Autodesk Inventor part; units mm, degrees
(part 2 of 4)
  spline S285 degree 3 poles (-158.7452, 2.7796) (-159.3519, 3.3863) (-159.5334, 4.2987) (-159.205, 5.0914) knots 0 0 0 0 1 1 1 1 construction
  spline S286 degree 3 poles (-159.205, 5.0914) (-158.8767, 5.8841) (-158.1032, 6.4009) (-157.2452, 6.4009) knots 0 0 0 0 1 1 1 1 construction
  arc A68 (-155.1239, 4.2796) -> (-157.2452, 6.4009) centre (-157.2452, 4.2796) ccw construction
  spline S287 degree 3 poles (-145.4719, 23.3296) (-145.4719, 22.4716) (-145.9887, 21.6981) (-146.7814, 21.3698) knots 0 0 0 0 1 1 1 1 construction
  spline S288 degree 3 poles (-146.7814, 21.3698) (-147.5741, 21.0414) (-148.4865, 21.2229) (-149.0932, 21.8296) knots 0 0 0 0 1 1 1 1 construction
  spline S289 degree 3 poles (-149.0932, 21.8296) (-149.6999, 22.4363) (-149.8814, 23.3487) (-149.553, 24.1414) knots 0 0 0 0 1 1 1 1 construction
  spline S290 degree 3 poles (-149.553, 24.1414) (-149.2247, 24.9341) (-148.4512, 25.4509) (-147.5932, 25.4509) knots 0 0 0 0 1 1 1 1 construction
  arc A69 (-145.4719, 23.3296) -> (-147.5932, 25.4509) centre (-147.5932, 23.3296) ccw construction
  spline S291 degree 3 poles (-136.0739, 4.2796) (-136.0739, 3.4216) (-136.5907, 2.6481) (-137.3834, 2.3198) knots 0 0 0 0 1 1 1 1 construction
  spline S292 degree 3 poles (-137.3834, 2.3198) (-138.1761, 1.9914) (-139.0885, 2.1729) (-139.6952, 2.7796) knots 0 0 0 0 1 1 1 1 construction
  spline S293 degree 3 poles (-139.6952, 2.7796) (-140.3019, 3.3863) (-140.4834, 4.2987) (-140.155, 5.0914) knots 0 0 0 0 1 1 1 1 construction
  spline S294 degree 3 poles (-140.155, 5.0914) (-139.8267, 5.8841) (-139.0532, 6.4009) (-138.1952, 6.4009) knots 0 0 0 0 1 1 1 1 construction
  arc A70 (-136.0739, 4.2796) -> (-138.1952, 6.4009) centre (-138.1952, 4.2796) ccw construction
  spline S295 degree 3 poles (-140.6459, -33.8204) (-140.6459, -34.6784) (-141.1627, -35.4519) (-141.9554, -35.7802) knots 0 0 0 0 1 1 1 1 construction
  spline S296 degree 3 poles (-141.9554, -35.7802) (-142.7481, -36.1086) (-143.6605, -35.9271) (-144.2672, -35.3204) knots 0 0 0 0 1 1 1 1 construction
  spline S297 degree 3 poles (-144.2672, -35.3204) (-144.8739, -34.7137) (-145.0554, -33.8013) (-144.727, -33.0086) knots 0 0 0 0 1 1 1 1 construction
  spline S298 degree 3 poles (-144.727, -33.0086) (-144.3987, -32.2159) (-143.6252, -31.6991) (-142.7672, -31.6991) knots 0 0 0 0 1 1 1 1 construction
  arc A71 (-140.6459, -33.8204) -> (-142.7672, -31.6991) centre (-142.7672, -33.8204) ccw construction
  spline S299 degree 3 poles (-131.2479, -14.7704) (-131.2479, -15.6284) (-131.7647, -16.4019) (-132.5574, -16.7302) knots 0 0 0 0 1 1 1 1 construction
  spline S300 degree 3 poles (-132.5574, -16.7302) (-133.3501, -17.0586) (-134.2625, -16.8771) (-134.8692, -16.2704) knots 0 0 0 0 1 1 1 1 construction
  spline S301 degree 3 poles (-134.8692, -16.2704) (-135.4759, -15.6637) (-135.6574, -14.7513) (-135.329, -13.9586) knots 0 0 0 0 1 1 1 1 construction
  spline S302 degree 3 poles (-135.329, -13.9586) (-135.0007, -13.1659) (-134.2272, -12.6491) (-133.3692, -12.6491) knots 0 0 0 0 1 1 1 1 construction
  arc A72 (-131.2479, -14.7704) -> (-133.3692, -12.6491) centre (-133.3692, -14.7704) ccw construction
  spline S303 degree 3 poles (-121.5959, -33.8204) (-121.5959, -34.6784) (-122.1127, -35.4519) (-122.9054, -35.7802) knots 0 0 0 0 1 1 1 1 construction
  spline S304 degree 3 poles (-122.9054, -35.7802) (-123.6981, -36.1086) (-124.6105, -35.9271) (-125.2172, -35.3204) knots 0 0 0 0 1 1 1 1 construction
  spline S305 degree 3 poles (-125.2172, -35.3204) (-125.8239, -34.7137) (-126.0054, -33.8013) (-125.677, -33.0086) knots 0 0 0 0 1 1 1 1 construction
  spline S306 degree 3 poles (-125.677, -33.0086) (-125.3487, -32.2159) (-124.5752, -31.6991) (-123.7172, -31.6991) knots 0 0 0 0 1 1 1 1 construction
  arc A73 (-121.5959, -33.8204) -> (-123.7172, -31.6991) centre (-123.7172, -33.8204) ccw construction
  arc A74 (-102.5459, -33.8204) -> (-104.6672, -31.6991) centre (-104.6672, -33.8204) ccw construction
  spline S307 degree 3 poles (-102.5459, -33.8204) (-102.5459, -34.6784) (-103.0627, -35.4519) (-103.8554, -35.7802) knots 0 0 0 0 1 1 1 1 construction
  spline S308 degree 3 poles (-103.8554, -35.7802) (-104.6481, -36.1086) (-105.5605, -35.9271) (-106.1672, -35.3204) knots 0 0 0 0 1 1 1 1 construction
  spline S309 degree 3 poles (-106.1672, -35.3204) (-106.7739, -34.7137) (-106.9554, -33.8013) (-106.627, -33.0086) knots 0 0 0 0 1 1 1 1 construction
  spline S310 degree 3 poles (-106.627, -33.0086) (-106.2987, -32.2159) (-105.5252, -31.6991) (-104.6672, -31.6991) knots 0 0 0 0 1 1 1 1 construction
  spline S311 degree 3 poles (-112.1979, -14.7704) (-112.1979, -15.6284) (-112.7147, -16.4019) (-113.5074, -16.7302) knots 0 0 0 0 1 1 1 1 construction
  spline S312 degree 3 poles (-113.5074, -16.7302) (-114.3001, -17.0586) (-115.2125, -16.8771) (-115.8192, -16.2704) knots 0 0 0 0 1 1 1 1 construction
  spline S313 degree 3 poles (-115.8192, -16.2704) (-116.4259, -15.6637) (-116.6074, -14.7513) (-116.279, -13.9586) knots 0 0 0 0 1 1 1 1 construction
  spline S314 degree 3 poles (-116.279, -13.9586) (-115.9507, -13.1659) (-115.1772, -12.6491) (-114.3192, -12.6491) knots 0 0 0 0 1 1 1 1 construction
  arc A75 (-112.1979, -14.7704) -> (-114.3192, -12.6491) centre (-114.3192, -14.7704) ccw construction
  line L28 (-145.8754, -43.9454) -> (-139.8754, -43.9454) construction
  line L29 (-139.8754, -43.9454) -> (-139.8754, -58.9454) construction
  line L30 (-139.8754, -58.9454) -> (-145.8754, -58.9454) construction
  line L31 (-145.8754, -58.9454) -> (-145.8754, -43.9454) construction
  spline S315 degree 3 poles (-134.5894, 49.9986) (-135.3821, 49.6702) (-136.2945, 49.8517) (-136.9012, 50.4584) knots 0 0 0 0 1 1 1 1 construction
  spline S316 degree 3 poles (-136.9012, 50.4584) (-137.5079, 51.0651) (-137.6894, 51.9775) (-137.361, 52.7702) knots 0 0 0 0 1 1 1 1 construction
  spline S317 degree 3 poles (-137.361, 52.7702) (-137.0327, 53.5629) (-136.2592, 54.0797) (-135.4012, 54.0797) knots 0 0 0 0 1 1 1 1 construction
  arc A76 (-133.2799, 51.9584) -> (-135.4012, 54.0797) centre (-135.4012, 51.9584) ccw construction
  spline S318 degree 3 poles (-133.2799, 51.9584) (-133.2799, 51.1004) (-133.7967, 50.3269) (-134.5894, 49.9986) knots 0 0 0 0 1 1 1 1 construction
  spline S319 degree 3 poles (-113.0252, 50.4864) (-113.6319, 51.0931) (-113.8134, 52.0055) (-113.485, 52.7982) knots 0 0 0 0 1 1 1 1 construction
  spline S320 degree 3 poles (-113.485, 52.7982) (-113.1567, 53.5909) (-112.3832, 54.1077) (-111.5252, 54.1077) knots 0 0 0 0 1 1 1 1 construction
  arc A77 (-109.4039, 51.9864) -> (-111.5252, 54.1077) centre (-111.5252, 51.9864) ccw construction
  spline S321 degree 3 poles (-109.4039, 51.9864) (-109.4039, 51.1284) (-109.9207, 50.3549) (-110.7134, 50.0266) knots 0 0 0 0 1 1 1 1 construction
  spline S322 degree 3 poles (-110.7134, 50.0266) (-111.5061, 49.6982) (-112.4185, 49.8797) (-113.0252, 50.4864) knots 0 0 0 0 1 1 1 1 construction
  arc A78 (-108.25, 37.6384) -> (-110, 39.3884) centre (-110, 37.6384) ccw construction
  spline S323 degree 3 poles (-108.25, 37.6384) (-108.25, 36.9306) (-108.6764, 36.2925) (-109.3303, 36.0216) knots 0 0 0 0 1 1 1 1 construction
  spline S324 degree 3 poles (-109.3303, 36.0216) (-109.9842, 35.7507) (-110.7369, 35.9005) (-111.2374, 36.401) knots 0 0 0 0 1 1 1 1 construction
  spline S325 degree 3 poles (-111.2374, 36.401) (-111.7379, 36.9015) (-111.8877, 37.6542) (-111.6168, 38.3081) knots 0 0 0 0 1 1 1 1 construction
  spline S326 degree 3 poles (-111.6168, 38.3081) (-111.3459, 38.962) (-110.7078, 39.3884) (-110, 39.3884) knots 0 0 0 0 1 1 1 1 construction
  arc A79 (-117.0239, 4.2796) -> (-119.1452, 6.4009) centre (-119.1452, 4.2796) ccw construction
  spline S327 degree 3 poles (-117.0239, 4.2796) (-117.0239, 3.4216) (-117.5407, 2.6481) (-118.3334, 2.3198) knots 0 0 0 0 1 1 1 1 construction
  spline S328 degree 3 poles (-118.3334, 2.3198) (-119.1261, 1.9914) (-120.0385, 2.1729) (-120.6452, 2.7796) knots 0 0 0 0 1 1 1 1 construction
  spline S329 degree 3 poles (-120.6452, 2.7796) (-121.2519, 3.3863) (-121.4334, 4.2987) (-121.105, 5.0914) knots 0 0 0 0 1 1 1 1 construction
  spline S330 degree 3 poles (-121.105, 5.0914) (-120.7767, 5.8841) (-120.0032, 6.4009) (-119.1452, 6.4009) knots 0 0 0 0 1 1 1 1 construction
  arc A80 (-107.3719, 23.3296) -> (-109.4932, 25.4509) centre (-109.4932, 23.3296) ccw construction
  spline S331 degree 3 poles (-107.3719, 23.3296) (-107.3719, 22.4716) (-107.8887, 21.6981) (-108.6814, 21.3698) knots 0 0 0 0 1 1 1 1 construction
  spline S332 degree 3 poles (-108.6814, 21.3698) (-109.4741, 21.0414) (-110.3865, 21.2229) (-110.9932, 21.8296) knots 0 0 0 0 1 1 1 1 construction
  spline S333 degree 3 poles (-110.9932, 21.8296) (-111.5999, 22.4363) (-111.7814, 23.3487) (-111.453, 24.1414) knots 0 0 0 0 1 1 1 1 construction
  spline S334 degree 3 poles (-111.453, 24.1414) (-111.1247, 24.9341) (-110.3512, 25.4509) (-109.4932, 25.4509) knots 0 0 0 0 1 1 1 1 construction
  arc A81 (-126.4219, 23.3296) -> (-128.5432, 25.4509) centre (-128.5432, 23.3296) ccw construction
  spline S335 degree 3 poles (-126.4219, 23.3296) (-126.4219, 22.158) (-127.3716, 21.2083) (-128.5432, 21.2083) knots 0 0 0 0 1 1 1 1 construction
  spline S336 degree 3 poles (-128.5432, 21.2083) (-129.7148, 21.2083) (-130.6645, 22.158) (-130.6645, 23.3296) knots 0 0 0 0 1 1 1 1 construction
  spline S337 degree 3 poles (-130.6645, 23.3296) (-130.6645, 24.5012) (-129.7148, 25.4509) (-128.5432, 25.4509) knots 0 0 0 0 1 1 1 1 construction
  arc A82 (-97.9739, 4.2008) -> (-100.0952, 6.3221) centre (-100.0952, 4.2008) ccw construction
  spline S338 degree 3 poles (-97.9739, 4.2008) (-97.9739, 3.3428) (-98.4907, 2.5693) (-99.2834, 2.241) knots 0 0 0 0 1 1 1 1 construction
  spline S339 degree 3 poles (-99.2834, 2.241) (-100.0761, 1.9126) (-100.9885, 2.0941) (-101.5952, 2.7008) knots 0 0 0 0 1 1 1 1 construction
  spline S340 degree 3 poles (-101.5952, 2.7008) (-102.2019, 3.3075) (-102.3834, 4.2199) (-102.055, 5.0126) knots 0 0 0 0 1 1 1 1 construction
  spline S341 degree 3 poles (-102.055, 5.0126) (-101.7267, 5.8053) (-100.9532, 6.3221) (-100.0952, 6.3221) knots 0 0 0 0 1 1 1 1 construction
  spline S342 degree 3 poles (-108.25, -57.5) (-108.25, -58.2078) (-108.6764, -58.8459) (-109.3303, -59.1168) knots 0 0 0 0 1 1 1 1 construction
  spline S343 degree 3 poles (-109.3303, -59.1168) (-109.9842, -59.3877) (-110.7369, -59.2379) (-111.2374, -58.7374) knots 0 0 0 0 1 1 1 1 construction
  spline S344 degree 3 poles (-111.2374, -58.7374) (-111.7379, -58.2369) (-111.8877, -57.4842) (-111.6168, -56.8303) knots 0 0 0 0 1 1 1 1 construction
  spline S345 degree 3 poles (-111.6168, -56.8303) (-111.3459, -56.1764) (-110.7078, -55.75) (-110, -55.75) knots 0 0 0 0 1 1 1 1 construction
  arc A83 (-108.25, -57.5) -> (-110, -55.75) centre (-110, -57.5) ccw construction
  spline S346 degree 3 poles (-93.1479, -14.7704) (-93.1479, -15.6284) (-93.6647, -16.4019) (-94.4574, -16.7302) knots 0 0 0 0 1 1 1 1 construction
  spline S347 degree 3 poles (-94.4574, -16.7302) (-95.2501, -17.0586) (-96.1625, -16.8771) (-96.7692, -16.2704) knots 0 0 0 0 1 1 1 1 construction
  spline S348 degree 3 poles (-96.7692, -16.2704) (-97.3759, -15.6637) (-97.5574, -14.7513) (-97.229, -13.9586) knots 0 0 0 0 1 1 1 1 construction
  spline S349 degree 3 poles (-97.229, -13.9586) (-96.9007, -13.1659) (-96.1272, -12.6491) (-95.2692, -12.6491) knots 0 0 0 0 1 1 1 1 construction
  spline S350 degree 3 poles (-95.2692, -12.6491) (-94.0976, -12.6491) (-93.1479, -13.5988) (-93.1479, -14.7704) knots 0 0 0 0 1 1 1 1 construction
  spline S351 degree 3 poles (-83.4959, -33.8204) (-83.4959, -34.6784) (-84.0127, -35.4519) (-84.8054, -35.7802) knots 0 0 0 0 1 1 1 1 construction
  spline S352 degree 3 poles (-84.8054, -35.7802) (-85.5981, -36.1086) (-86.5105, -35.9271) (-87.1172, -35.3204) knots 0 0 0 0 1 1 1 1 construction
  spline S353 degree 3 poles (-87.1172, -35.3204) (-87.7239, -34.7137) (-87.9054, -33.8013) (-87.577, -33.0086) knots 0 0 0 0 1 1 1 1 construction
  spline S354 degree 3 poles (-87.577, -33.0086) (-87.2487, -32.2159) (-86.4752, -31.6991) (-85.6172, -31.6991) knots 0 0 0 0 1 1 1 1 construction
  spline S355 degree 3 poles (-85.6172, -31.6991) (-84.4456, -31.6991) (-83.4959, -32.6488) (-83.4959, -33.8204) knots 0 0 0 0 1 1 1 1 construction
  spline S356 degree 3 poles (-89.1492, 50.4864) (-89.7559, 51.0931) (-89.9374, 52.0055) (-89.609, 52.7982) knots 0 0 0 0 1 1 1 1 construction
  spline S357 degree 3 poles (-89.609, 52.7982) (-89.2807, 53.5909) (-88.5072, 54.1077) (-87.6492, 54.1077) knots 0 0 0 0 1 1 1 1 construction
  arc A84 (-85.5279, 51.9864) -> (-87.6492, 54.1077) centre (-87.6492, 51.9864) ccw construction
  spline S358 degree 3 poles (-85.5279, 51.9864) (-85.5279, 51.1284) (-86.0447, 50.3549) (-86.8374, 50.0266) knots 0 0 0 0 1 1 1 1 construction
  spline S359 degree 3 poles (-86.8374, 50.0266) (-87.6301, 49.6982) (-88.5425, 49.8797) (-89.1492, 50.4864) knots 0 0 0 0 1 1 1 1 construction
  spline S360 degree 3 poles (-56.6432, 50.4864) (-57.2499, 51.0931) (-57.4314, 52.0055) (-57.103, 52.7982) knots 0 0 0 0 1 1 1 1 construction
  spline S361 degree 3 poles (-57.103, 52.7982) (-56.7747, 53.5909) (-56.0012, 54.1077) (-55.1432, 54.1077) knots 0 0 0 0 1 1 1 1 construction
  arc A85 (-53.0219, 51.9864) -> (-55.1432, 54.1077) centre (-55.1432, 51.9864) ccw construction
  spline S362 degree 3 poles (-53.0219, 51.9864) (-53.0219, 51.1284) (-53.5387, 50.3549) (-54.3314, 50.0266) knots 0 0 0 0 1 1 1 1 construction
  spline S363 degree 3 poles (-54.3314, 50.0266) (-55.1241, 49.6982) (-56.0365, 49.8797) (-56.6432, 50.4864) knots 0 0 0 0 1 1 1 1 construction
  spline S364 degree 3 poles (-72.8932, 21.8296) (-73.4999, 22.4363) (-73.6814, 23.3487) (-73.353, 24.1414) knots 0 0 0 0 1 1 1 1 construction
  spline S365 degree 3 poles (-73.353, 24.1414) (-73.0247, 24.9341) (-72.2512, 25.4509) (-71.3932, 25.4509) knots 0 0 0 0 1 1 1 1 construction
  arc A86 (-69.2719, 23.3296) -> (-71.3932, 25.4509) centre (-71.3932, 23.3296) ccw construction
  spline S366 degree 3 poles (-69.2719, 23.3296) (-69.2719, 22.4716) (-69.7887, 21.6981) (-70.5814, 21.3698) knots 0 0 0 0 1 1 1 1 construction
  spline S367 degree 3 poles (-70.5814, 21.3698) (-71.3741, 21.0414) (-72.2865, 21.2229) (-72.8932, 21.8296) knots 0 0 0 0 1 1 1 1 construction
  spline S368 degree 3 poles (-53.8432, 21.8296) (-54.4499, 22.4363) (-54.6314, 23.3487) (-54.303, 24.1414) knots 0 0 0 0 1 1 1 1 construction
  spline S369 degree 3 poles (-54.303, 24.1414) (-53.9747, 24.9341) (-53.2012, 25.4509) (-52.3432, 25.4509) knots 0 0 0 0 1 1 1 1 construction
  arc A87 (-50.2219, 23.3296) -> (-52.3432, 25.4509) centre (-52.3432, 23.3296) ccw construction
  spline S370 degree 3 poles (-50.2219, 23.3296) (-50.2219, 22.4716) (-50.7387, 21.6981) (-51.5314, 21.3698) knots 0 0 0 0 1 1 1 1 construction
  spline S371 degree 3 poles (-51.5314, 21.3698) (-52.3241, 21.0414) (-53.2365, 21.2229) (-53.8432, 21.8296) knots 0 0 0 0 1 1 1 1 construction
  spline S372 degree 3 poles (-88.3219, 23.3296) (-88.3219, 22.4716) (-88.8387, 21.6981) (-89.6314, 21.3698) knots 0 0 0 0 1 1 1 1 construction
  spline S373 degree 3 poles (-89.6314, 21.3698) (-90.4241, 21.0414) (-91.3365, 21.2229) (-91.9432, 21.8296) knots 0 0 0 0 1 1 1 1 construction
  spline S374 degree 3 poles (-91.9432, 21.8296) (-92.5499, 22.4363) (-92.7314, 23.3487) (-92.403, 24.1414) knots 0 0 0 0 1 1 1 1 construction
  spline S375 degree 3 poles (-92.403, 24.1414) (-92.0747, 24.9341) (-91.3012, 25.4509) (-90.4432, 25.4509) knots 0 0 0 0 1 1 1 1 construction
  spline S376 degree 3 poles (-90.4432, 25.4509) (-89.2716, 25.4509) (-88.3219, 24.5012) (-88.3219, 23.3296) knots 0 0 0 0 1 1 1 1 construction
  spline S377 degree 3 poles (-59.129, -13.9586) (-58.8007, -13.1659) (-58.0272, -12.6491) (-57.1692, -12.6491) knots 0 0 0 0 1 1 1 1 construction
  arc A88 (-55.0479, -14.7704) -> (-57.1692, -12.6491) centre (-57.1692, -14.7704) ccw construction
  spline S378 degree 3 poles (-55.0479, -14.7704) (-55.0479, -15.6284) (-55.5647, -16.4019) (-56.3574, -16.7302) knots 0 0 0 0 1 1 1 1 construction
  spline S379 degree 3 poles (-56.3574, -16.7302) (-57.1501, -17.0586) (-58.0625, -16.8771) (-58.6692, -16.2704) knots 0 0 0 0 1 1 1 1 construction
  spline S380 degree 3 poles (-58.6692, -16.2704) (-59.2759, -15.6637) (-59.4574, -14.7513) (-59.129, -13.9586) knots 0 0 0 0 1 1 1 1 construction
  spline S381 degree 3 poles (-68.527, -33.0086) (-68.1987, -32.2159) (-67.4252, -31.6991) (-66.5672, -31.6991) knots 0 0 0 0 1 1 1 1 construction
  arc A89 (-64.4459, -33.8204) -> (-66.5672, -31.6991) centre (-66.5672, -33.8204) ccw construction
  spline S382 degree 3 poles (-64.4459, -33.8204) (-64.4459, -34.6784) (-64.9627, -35.4519) (-65.7554, -35.7802) knots 0 0 0 0 1 1 1 1 construction
  spline S383 degree 3 poles (-65.7554, -35.7802) (-66.5481, -36.1086) (-67.4605, -35.9271) (-68.0672, -35.3204) knots 0 0 0 0 1 1 1 1 construction
  spline S384 degree 3 poles (-68.0672, -35.3204) (-68.6739, -34.7137) (-68.8554, -33.8013) (-68.527, -33.0086) knots 0 0 0 0 1 1 1 1 construction
  spline S385 degree 3 poles (-78.179, -13.9586) (-77.8507, -13.1659) (-77.0772, -12.6491) (-76.2192, -12.6491) knots 0 0 0 0 1 1 1 1 construction
  arc A90 (-74.0979, -14.7704) -> (-76.2192, -12.6491) centre (-76.2192, -14.7704) ccw construction
  spline S386 degree 3 poles (-74.0979, -14.7704) (-74.0979, -15.6284) (-74.6147, -16.4019) (-75.4074, -16.7302) knots 0 0 0 0 1 1 1 1 construction
  spline S387 degree 3 poles (-75.4074, -16.7302) (-76.2001, -17.0586) (-77.1125, -16.8771) (-77.7192, -16.2704) knots 0 0 0 0 1 1 1 1 construction
  spline S388 degree 3 poles (-77.7192, -16.2704) (-78.3259, -15.6637) (-78.5074, -14.7513) (-78.179, -13.9586) knots 0 0 0 0 1 1 1 1 construction
  arc A91 (-45.3959, -33.8204) -> (-47.5172, -31.6991) centre (-47.5172, -33.8204) ccw construction
  spline S389 degree 3 poles (-45.3959, -33.8204) (-45.3959, -34.6784) (-45.9127, -35.4519) (-46.7054, -35.7802) knots 0 0 0 0 1 1 1 1 construction
  spline S390 degree 3 poles (-46.7054, -35.7802) (-47.4981, -36.1086) (-48.4105, -35.9271) (-49.0172, -35.3204) knots 0 0 0 0 1 1 1 1 construction
  spline S391 degree 3 poles (-49.0172, -35.3204) (-49.6239, -34.7137) (-49.8054, -33.8013) (-49.477, -33.0086) knots 0 0 0 0 1 1 1 1 construction
  spline S392 degree 3 poles (-49.477, -33.0086) (-49.1487, -32.2159) (-48.3752, -31.6991) (-47.5172, -31.6991) knots 0 0 0 0 1 1 1 1 construction
  arc A92 (-74.6059, -52.8704) -> (-76.7272, -50.7491) centre (-76.7272, -52.8704) ccw construction
  spline S393 degree 3 poles (-74.6059, -52.8704) (-74.6059, -53.7284) (-75.1227, -54.5019) (-75.9154, -54.8302) knots 0 0 0 0 1 1 1 1 construction
  spline S394 degree 3 poles (-75.9154, -54.8302) (-76.7081, -55.1586) (-77.6205, -54.9771) (-78.2272, -54.3704) knots 0 0 0 0 1 1 1 1 construction
  spline S395 degree 3 poles (-78.2272, -54.3704) (-78.8339, -53.7637) (-79.0154, -52.8513) (-78.687, -52.0586) knots 0 0 0 0 1 1 1 1 construction
  spline S396 degree 3 poles (-78.687, -52.0586) (-78.3587, -51.2659) (-77.5852, -50.7491) (-76.7272, -50.7491) knots 0 0 0 0 1 1 1 1 construction
  arc A93 (-59.8739, 4.2796) -> (-61.9952, 6.4009) centre (-61.9952, 4.2796) ccw construction
  spline S397 degree 3 poles (-59.8739, 4.2796) (-59.8739, 3.4216) (-60.3907, 2.6481) (-61.1834, 2.3198) knots 0 0 0 0 1 1 1 1 construction
  spline S398 degree 3 poles (-61.1834, 2.3198) (-61.9761, 1.9914) (-62.8885, 2.1729) (-63.4952, 2.7796) knots 0 0 0 0 1 1 1 1 construction
  spline S399 degree 3 poles (-63.4952, 2.7796) (-64.1019, 3.3863) (-64.2834, 4.2987) (-63.955, 5.0914) knots 0 0 0 0 1 1 1 1 construction
  spline S400 degree 3 poles (-63.955, 5.0914) (-63.6267, 5.8841) (-62.8532, 6.4009) (-61.9952, 6.4009) knots 0 0 0 0 1 1 1 1 construction
  arc A94 (-78.9239, 4.2796) -> (-81.0452, 6.4009) centre (-81.0452, 4.2796) ccw construction
  spline S401 degree 3 poles (-78.9239, 4.2796) (-78.9239, 3.4216) (-79.4407, 2.6481) (-80.2334, 2.3198) knots 0 0 0 0 1 1 1 1 construction
  spline S402 degree 3 poles (-80.2334, 2.3198) (-81.0261, 1.9914) (-81.9385, 2.1729) (-82.5452, 2.7796) knots 0 0 0 0 1 1 1 1 construction
  spline S403 degree 3 poles (-82.5452, 2.7796) (-83.1519, 3.3863) (-83.3334, 4.2987) (-83.005, 5.0914) knots 0 0 0 0 1 1 1 1 construction
  spline S404 degree 3 poles (-83.005, 5.0914) (-82.6767, 5.8841) (-81.9032, 6.4009) (-81.0452, 6.4009) knots 0 0 0 0 1 1 1 1 construction
  arc A95 (-40.8239, 4.2796) -> (-42.9452, 6.4009) centre (-42.9452, 4.2796) ccw construction
  spline S405 degree 3 poles (-40.8239, 4.2796) (-40.8239, 3.4216) (-41.3407, 2.6481) (-42.1334, 2.3198) knots 0 0 0 0 1 1 1 1 construction
  spline S406 degree 3 poles (-42.1334, 2.3198) (-42.9261, 1.9914) (-43.8385, 2.1729) (-44.4452, 2.7796) knots 0 0 0 0 1 1 1 1 construction
  spline S407 degree 3 poles (-44.4452, 2.7796) (-45.0519, 3.3863) (-45.2334, 4.2987) (-44.905, 5.0914) knots 0 0 0 0 1 1 1 1 construction
  spline S408 degree 3 poles (-44.905, 5.0914) (-44.5767, 5.8841) (-43.8032, 6.4009) (-42.9452, 6.4009) knots 0 0 0 0 1 1 1 1 construction
  spline S409 degree 3 poles (219.7443, 55.7135) (220.682, 54.7759) (221.2088, 53.5041) (221.2088, 52.178) knots 0 0 0 0 1 1 1 1 construction
  spline S410 degree 3 poles (221.2088, 52.178) (221.2088, 50.1557) (219.9906, 48.3325) (218.1222, 47.5586) knots 0 0 0 0 1 1 1 1 construction
  spline S411 degree 3 poles (218.1222, 47.5586) (216.2538, 46.7847) (214.1033, 47.2125) (212.6733, 48.6425) knots 0 0 0 0 1 1 1 1 construction
  spline S412 degree 3 poles (212.6733, 48.6425) (211.2433, 50.0725) (210.8155, 52.223) (211.5894, 54.0914) knots 0 0 0 0 1 1 1 1 construction
  spline S413 degree 3 poles (211.5894, 54.0914) (212.3633, 55.9598) (214.1865, 57.178) (216.2088, 57.178) knots 0 0 0 0 1 1 1 1 construction
  spline S414 degree 3 poles (216.2088, 57.178) (217.5349, 57.178) (218.8067, 56.6512) (219.7443, 55.7135) knots 0 0 0 0 1 1 1 1 construction
  line L32 (204.7088, -52.274) -> (219.7088, -52.274) construction
  line L33 (219.7088, -52.274) -> (219.7088, -58.274) construction
  line L34 (219.7088, -58.274) -> (204.7088, -58.274) construction
  line L35 (204.7088, -58.274) -> (204.7088, -52.274) construction
  spline S415 degree 3 poles (218.3832, 38.3081) (218.6541, 38.962) (219.2922, 39.3884) (220, 39.3884) knots 0 0 0 0 1 1 1 1 construction
  arc A96 (221.75, 37.6384) -> (220, 39.3884) centre (220, 37.6384) ccw construction
  spline S416 degree 3 poles (221.75, 37.6384) (221.75, 36.9306) (221.3236, 36.2925) (220.6697, 36.0216) knots 0 0 0 0 1 1 1 1 construction
  spline S417 degree 3 poles (220.6697, 36.0216) (220.0158, 35.7507) (219.2631, 35.9005) (218.7626, 36.401) knots 0 0 0 0 1 1 1 1 construction
  spline S418 degree 3 poles (218.7626, 36.401) (218.2621, 36.9015) (218.1123, 37.6542) (218.3832, 38.3081) knots 0 0 0 0 1 1 1 1 construction
  spline S419 degree 3 poles (146.9023, 58.0219) (147.84, 57.0843) (148.3668, 55.8125) (148.3668, 54.4864) knots 0 0 0 0 1 1 1 1 construction
  spline S420 degree 3 poles (148.3668, 54.4864) (148.3668, 52.4641) (147.1486, 50.6409) (145.2802, 49.867) knots 0 0 0 0 1 1 1 1 construction
  spline S421 degree 3 poles (145.2802, 49.867) (143.4118, 49.0931) (141.2613, 49.5209) (139.8313, 50.9509) knots 0 0 0 0 1 1 1 1 construction
  spline S422 degree 3 poles (139.8313, 50.9509) (138.4013, 52.3809) (137.9735, 54.5314) (138.7474, 56.3998) knots 0 0 0 0 1 1 1 1 construction
  spline S423 degree 3 poles (138.7474, 56.3998) (139.5213, 58.2682) (141.3445, 59.4864) (143.3668, 59.4864) knots 0 0 0 0 1 1 1 1 construction
  spline S424 degree 3 poles (143.3668, 59.4864) (144.6929, 59.4864) (145.9647, 58.9596) (146.9023, 58.0219) knots 0 0 0 0 1 1 1 1 construction
  arc A97 (111.75, 37.6384) -> (110, 39.3884) centre (110, 37.6384) ccw construction
  spline S425 degree 3 poles (111.75, 37.6384) (111.75, 36.9306) (111.3236, 36.2925) (110.6697, 36.0216) knots 0 0 0 0 1 1 1 1 construction
  spline S426 degree 3 poles (110.6697, 36.0216) (110.0158, 35.7507) (109.2631, 35.9005) (108.7626, 36.401) knots 0 0 0 0 1 1 1 1 construction
  spline S427 degree 3 poles (108.7626, 36.401) (108.2621, 36.9015) (108.1123, 37.6542) (108.3832, 38.3081) knots 0 0 0 0 1 1 1 1 construction
  spline S428 degree 3 poles (108.3832, 38.3081) (108.6541, 38.962) (109.2922, 39.3884) (110, 39.3884) knots 0 0 0 0 1 1 1 1 construction
  spline S429 degree 3 poles (47.5681, -33.8204) (47.5681, -34.6784) (47.0513, -35.4519) (46.2586, -35.7802) knots 0 0 0 0 1 1 1 1 construction
  spline S430 degree 3 poles (46.2586, -35.7802) (45.4659, -36.1086) (44.5535, -35.9271) (43.9468, -35.3204) knots 0 0 0 0 1 1 1 1 construction
  spline S431 degree 3 poles (43.9468, -35.3204) (43.3401, -34.7137) (43.1586, -33.8013) (43.487, -33.0086) knots 0 0 0 0 1 1 1 1 construction
  spline S432 degree 3 poles (43.487, -33.0086) (43.8153, -32.2159) (44.5888, -31.6991) (45.4468, -31.6991) knots 0 0 0 0 1 1 1 1 construction
  arc A98 (47.5681, -33.8204) -> (45.4468, -31.6991) centre (45.4468, -33.8204) ccw construction
  spline S433 degree 3 poles (218.3832, -23.8303) (218.6541, -23.1764) (219.2922, -22.75) (220, -22.75) knots 0 0 0 0 1 1 1 1 construction
  arc A99 (221.75, -24.5) -> (220, -22.75) centre (220, -24.5) ccw construction
  spline S434 degree 3 poles (221.75, -24.5) (221.75, -25.2078) (221.3236, -25.8459) (220.6697, -26.1168) knots 0 0 0 0 1 1 1 1 construction
  spline S435 degree 3 poles (220.6697, -26.1168) (220.0158, -26.3877) (219.2631, -26.2379) (218.7626, -25.7374) knots 0 0 0 0 1 1 1 1 construction
  spline S436 degree 3 poles (218.7626, -25.7374) (218.2621, -25.2369) (218.1123, -24.4842) (218.3832, -23.8303) knots 0 0 0 0 1 1 1 1 construction
  line L36 (204.7088, -28.274) -> (219.7088, -28.274) construction
  line L37 (219.7088, -28.274) -> (219.7088, -34.274) construction
  line L38 (219.7088, -34.274) -> (204.7088, -34.274) construction
  line L39 (204.7088, -34.274) -> (204.7088, -28.274) construction
  line L40 (151.2108, -58.772) -> (151.2108, -43.772) construction
  line L41 (151.2108, -43.772) -> (157.2108, -43.772) construction
  line L42 (157.2108, -43.772) -> (157.2108, -58.772) construction
  line L43 (157.2108, -58.772) -> (151.2108, -58.772) construction
  line L44 (175.2108, -58.772) -> (175.2108, -43.772) construction
  line L45 (175.2108, -43.772) -> (181.2108, -43.772) construction
  line L46 (181.2108, -43.772) -> (181.2108, -58.772) construction
  line L47 (181.2108, -58.772) -> (175.2108, -58.772) construction
  spline S437 degree 3 poles (191.7443, 55.7135) (192.682, 54.7759) (193.2088, 53.5041) (193.2088, 52.178) knots 0 0 0 0 1 1 1 1 construction
  spline S438 degree 3 poles (193.2088, 52.178) (193.2088, 50.1557) (191.9906, 48.3325) (190.1222, 47.5586) knots 0 0 0 0 1 1 1 1 construction
  spline S439 degree 3 poles (190.1222, 47.5586) (188.2538, 46.7847) (186.1033, 47.2125) (184.6733, 48.6425) knots 0 0 0 0 1 1 1 1 construction
  spline S440 degree 3 poles (184.6733, 48.6425) (183.2433, 50.0725) (182.8155, 52.223) (183.5894, 54.0914) knots 0 0 0 0 1 1 1 1 construction
  spline S441 degree 3 poles (183.5894, 54.0914) (184.3633, 55.9598) (186.1865, 57.178) (188.2088, 57.178) knots 0 0 0 0 1 1 1 1 construction
  spline S442 degree 3 poles (188.2088, 57.178) (189.5349, 57.178) (190.8067, 56.6512) (191.7443, 55.7135) knots 0 0 0 0 1 1 1 1 construction
  line L48 (65.6708, 3.6276) -> (50.6708, 3.6276) construction
  line L49 (50.6708, 3.6276) -> (50.6708, 9.6276) construction
  line L50 (50.6708, 9.6276) -> (65.6708, 9.6276) construction
  line L51 (65.6708, 9.6276) -> (65.6708, 3.6276) construction
  line L52 (4.4528, 42.3884) -> (4.4528, 61.3884) construction
  line L53 (4.4528, 37.558) -> (4.4528, 42.3884) construction
  line L54 (14.2318, 37.558) -> (4.4528, 37.558) construction
  line L55 (14.2318, 32.8296) -> (14.2318, 37.558) construction
  line L56 (14.2318, 13.9046) -> (14.2318, 32.8296) construction
  line L57 (4.4528, 13.9046) -> (14.2318, 13.9046) construction
  line L58 (4.4528, -5.3455) -> (4.4528, 13.9046) construction
  line L59 (9.6598, -5.3455) -> (4.4528, -5.3455) construction
  line L60 (9.6598, -24.1954) -> (9.6598, -5.3455) construction
  line L61 (0.0048, -24.1954) -> (9.6598, -24.1954) construction
  line L62 (0.0048, -49.2614) -> (0.0048, -24.1954) construction
  line L63 (8.4302, -49.2614) -> (0.0048, -49.2614) construction
  line L64 (8.4302, -62.3704) -> (8.4302, -49.2614) construction
  line L65 (4.5528, 62.5) -> (4.5528, 37.658) construction
  line L66 (4.5528, 37.658) -> (14.3318, 37.658) construction
  line L67 (14.3318, 37.658) -> (14.3318, 13.8046) construction
  line L68 (14.3318, 13.8046) -> (4.5528, 13.8046) construction
  line L69 (4.5528, 13.8046) -> (4.5528, -5.2455) construction
  line L70 (4.5528, -5.2455) -> (9.7598, -5.2455) construction
  line L71 (9.7598, -24.2954) -> (0.1048, -24.2954) construction
  line L72 (0.1048, -24.2954) -> (0.1048, -49.1614) construction
  line L73 (0.1048, -49.1614) -> (8.5302, -49.1614) construction
  line L74 (8.5302, -49.1614) -> (8.5302, -62.5) construction
  line L75 (9.7598, -5.2455) -> (9.7598, -24.2954) construction
  line L76 (4.6528, 62.5) -> (4.6528, 37.758) construction
  line L77 (4.6528, 37.758) -> (14.4318, 37.758)
  line L78 (14.4318, 37.758) -> (14.4318, 13.7046) construction
  line L79 (14.4318, 13.7046) -> (4.6528, 13.7046)
  line L80 (4.6528, 13.7046) -> (4.6528, -5.1455)
  line L81 (4.6528, -5.1455) -> (9.8598, -5.1455)
  line L82 (9.8598, -5.1455) -> (9.8598, -24.3954)
  line L83 (9.8598, -24.3954) -> (0.2048, -24.3954)
  line L84 (0.2048, -24.3954) -> (0.2048, -49.0614)
  line L85 (0.2048, -49.0614) -> (8.6302, -49.0614)
  line L86 (8.6302, -49.0614) -> (8.6302, -62.3704)
  line L87 (4.6528, 61.3884) -> (4.6528, 37.758)
  line L88 (14.4318, 37.758) -> (14.4318, 13.7046)
  line L89 (-209.6412, -62.3704) -> (57.4568, -62.3704) construction
  line L90 (-209.6412, -62.3704) -> (57.4568, -62.3704) construction
  line L91 (8.6302, -62.3704) -> (57.4568, -62.3704)
  line L92 (57.4568, -62.3704) -> (57.4568, -43.3204) projected
  line L93 (57.4568, -43.3204) -> (71.4568, -43.3204) projected
  line L94 (148.1338, -62.3704) -> (148.1338, 32.8296) construction
  line L95 (71.4568, -43.3204) -> (148.1338, -43.3204)
  line L96 (148.1338, -43.3204) -> (148.1338, -62.3704)
  line L97 (222.1338, -62.3704) -> (148.1338, -62.3704) projected
  line L98 (222.1338, 32.8296) -> (222.1338, -62.3704) projected
  line L99 (148.1338, 32.8296) -> (222.1338, 32.8296) construction
  line L100 (51.6148, 61.3884) -> (51.6148, 42.3884) construction
  line L101 (4.6528, 61.3884) -> (51.6148, 61.3884)
  line L102 (51.6148, 61.3884) -> (51.6148, 32.8296)
  line L103 (51.6148, 32.8296) -> (222.1338, 32.8296)
  line L104 (9.4883, 58.9889) -> (23.4933, 58.9889)
  line L105 (23.4933, 58.9889) -> (23.4933, 44.9839)
  line L106 (23.4933, 44.9839) -> (9.4883, 44.9839)
  line L107 (9.4883, 44.9839) -> (9.4883, 58.9889)
  line L108 (9.4883, 58.9889) -> (23.4933, 44.9839) construction
  line L109 (23.4933, 58.9889) -> (9.4883, 44.9839) construction
  line L110 (33.3643, 58.9889) -> (47.3693, 58.9889)
  line L111 (47.3693, 58.9889) -> (47.3693, 44.9839)
  line L112 (47.3693, 44.9839) -> (33.3643, 44.9839)
  line L113 (33.3643, 44.9839) -> (33.3643, 58.9889)
  line L114 (33.3643, 58.9889) -> (47.3693, 44.9839) construction
  line L115 (47.3693, 58.9889) -> (33.3643, 44.9839) construction
  line L116 (16.8543, 30.3321) -> (30.8593, 30.3321)
  line L117 (30.8593, 30.3321) -> (30.8593, 16.3271)
  line L118 (30.8593, 16.3271) -> (16.8543, 16.3271)
  line L119 (16.8543, 16.3271) -> (16.8543, 30.3321)
  line L120 (16.8543, 30.3321) -> (30.8593, 16.3271) construction
  line L121 (30.8593, 30.3321) -> (16.8543, 16.3271) construction
  line L122 (35.9043, 30.3321) -> (49.9093, 30.3321)
  line L123 (49.9093, 30.3321) -> (49.9093, 16.3271)
  line L124 (49.9093, 16.3271) -> (35.9043, 16.3271)
  line L125 (35.9043, 16.3271) -> (35.9043, 30.3321)
  line L126 (35.9043, 30.3321) -> (49.9093, 16.3271) construction
  line L127 (49.9093, 30.3321) -> (35.9043, 16.3271) construction
  line L128 (54.9543, 30.3321) -> (68.9593, 30.3321)
  line L129 (68.9593, 30.3321) -> (68.9593, 16.3271)
  line L130 (68.9593, 16.3271) -> (54.9543, 16.3271)
  line L131 (54.9543, 16.3271) -> (54.9543, 30.3321)
  line L132 (54.9543, 30.3321) -> (68.9593, 16.3271) construction
  line L133 (68.9593, 30.3321) -> (54.9543, 16.3271) construction
  line L134 (7.2023, 11.2821) -> (21.2073, 11.2821)
  line L135 (21.2073, 11.2821) -> (21.2073, -2.7229)
  line L136 (21.2073, -2.7229) -> (7.2023, -2.7229)
  line L137 (7.2023, -2.7229) -> (7.2023, 11.2821)
  line L138 (7.2023, 11.2821) -> (21.2073, -2.7229) construction
  line L139 (21.2073, 11.2821) -> (7.2023, -2.7229) construction
  line L140 (26.2523, 11.2821) -> (40.2573, 11.2821)
  line L141 (40.2573, 11.2821) -> (40.2573, -2.7229)
  line L142 (40.2573, -2.7229) -> (26.2523, -2.7229)
  line L143 (26.2523, -2.7229) -> (26.2523, 11.2821)
  line L144 (26.2523, 11.2821) -> (40.2573, -2.7229) construction
  line L145 (40.2573, 11.2821) -> (26.2523, -2.7229) construction
  line L146 (12.2823, -7.7679) -> (26.2873, -7.7679)
  line L147 (26.2873, -7.7679) -> (26.2873, -21.7729)
  line L148 (26.2873, -21.7729) -> (12.2823, -21.7729)
  line L149 (12.2823, -21.7729) -> (12.2823, -7.7679)
  line L150 (12.2823, -7.7679) -> (26.2873, -21.7729) construction
  line L151 (26.2873, -7.7679) -> (12.2823, -21.7729) construction
  line L152 (31.3323, -7.7679) -> (45.3373, -7.7679)
  line L153 (45.3373, -7.7679) -> (45.3373, -21.7729)
  line L154 (45.3373, -21.7729) -> (31.3323, -21.7729)
  line L155 (31.3323, -21.7729) -> (31.3323, -7.7679)
  line L156 (31.3323, -7.7679) -> (45.3373, -21.7729) construction
  line L157 (45.3373, -7.7679) -> (31.3323, -21.7729) construction
  line L158 (52.6683, 1.6301) -> (66.6733, 1.6301)
  line L159 (66.6733, 1.6301) -> (66.6733, -12.3749)
  line L160 (66.6733, -12.3749) -> (52.6683, -12.3749)
  line L161 (52.6683, -12.3749) -> (52.6683, 1.6301)
  line L162 (52.6683, 1.6301) -> (66.6733, -12.3749) construction
  line L163 (66.6733, 1.6301) -> (52.6683, -12.3749) construction
  line L164 (2.6303, -26.8179) -> (16.6353, -26.8179)
  line L165 (16.6353, -26.8179) -> (16.6353, -40.8229)
  line L166 (16.6353, -40.8229) -> (2.6303, -40.8229)
  line L167 (2.6303, -40.8229) -> (2.6303, -26.8179)
  line L168 (2.6303, -26.8179) -> (16.6353, -40.8229) construction
  line L169 (16.6353, -26.8179) -> (2.6303, -40.8229) construction
  line L170 (38.4443, -26.8179) -> (52.4493, -26.8179)
  line L171 (52.4493, -26.8179) -> (52.4493, -40.8229)
  line L172 (52.4493, -40.8229) -> (38.4443, -40.8229)
  line L173 (38.4443, -40.8229) -> (38.4443, -26.8179)
  line L174 (38.4443, -26.8179) -> (52.4493, -40.8229) construction
  line L175 (52.4493, -26.8179) -> (38.4443, -40.8229) construction
  line L176 (14.0603, -45.8679) -> (28.0653, -45.8679)
  line L177 (28.0653, -45.8679) -> (28.0653, -59.8729)
  line L178 (28.0653, -59.8729) -> (14.0603, -59.8729)
  line L179 (14.0603, -59.8729) -> (14.0603, -45.8679)
  line L180 (14.0603, -45.8679) -> (28.0653, -59.8729) construction
  line L181 (28.0653, -45.8679) -> (14.0603, -59.8729) construction
  line L182 (37.9363, -45.8679) -> (51.9413, -45.8679)
  line L183 (51.9413, -45.8679) -> (51.9413, -59.8729)
  line L184 (51.9413, -59.8729) -> (37.9363, -59.8729)
  line L185 (37.9363, -59.8729) -> (37.9363, -45.8679)
  line L186 (37.9363, -45.8679) -> (51.9413, -59.8729) construction
  line L187 (51.9413, -45.8679) -> (37.9363, -59.8729) construction
  line L188 (82.8275, -26.7671) -> (96.8325, -26.7671)
  line L189 (96.8325, -26.7671) -> (96.8325, -40.7721)
  line L190 (96.8325, -40.7721) -> (82.8275, -40.7721)
  line L191 (82.8275, -40.7721) -> (82.8275, -26.7671)
  line L192 (82.8275, -26.7671) -> (96.8325, -40.7721) construction
  line L193 (96.8325, -26.7671) -> (82.8275, -40.7721) construction
  line L194 (101.8775, -26.7671) -> (115.8825, -26.7671)
  line L195 (115.8825, -26.7671) -> (115.8825, -40.7721)
  line L196 (115.8825, -40.7721) -> (101.8775, -40.7721)
  line L197 (101.8775, -40.7721) -> (101.8775, -26.7671)
  line L198 (101.8775, -26.7671) -> (115.8825, -40.7721) construction
  line L199 (115.8825, -26.7671) -> (101.8775, -40.7721) construction
  line L200 (101.8775, -7.7171) -> (115.8825, -7.7171)
  line L201 (115.8825, -7.7171) -> (115.8825, -21.7221)
  line L202 (115.8825, -21.7221) -> (101.8775, -21.7221)
  line L203 (101.8775, -21.7221) -> (101.8775, -7.7171)
  line L204 (101.8775, -7.7171) -> (115.8825, -21.7221) construction
  line L205 (115.8825, -7.7171) -> (101.8775, -21.7221) construction
  line L206 (120.9275, -26.7671) -> (134.9325, -26.7671)
  line L207 (134.9325, -26.7671) -> (134.9325, -40.7721)
  line L208 (134.9325, -40.7721) -> (120.9275, -40.7721)
  line L209 (120.9275, -40.7721) -> (120.9275, -26.7671)
  line L210 (120.9275, -26.7671) -> (134.9325, -40.7721) construction
  line L211 (134.9325, -26.7671) -> (120.9275, -40.7721) construction
  line L212 (116.1515, 30.3969) -> (130.1565, 30.3969)
  line L213 (130.1565, 30.3969) -> (130.1565, 16.3919)
  line L214 (130.1565, 16.3919) -> (116.1515, 16.3919)
  line L215 (116.1515, 16.3919) -> (116.1515, 30.3969)
  line L216 (116.1515, 30.3969) -> (130.1565, 16.3919) construction
  line L217 (130.1565, 30.3969) -> (116.1515, 16.3919) construction
  line L218 (87.5555, 30.3969) -> (101.5605, 30.3969)
  line L219 (101.5605, 30.3969) -> (101.5605, 16.3919)
  line L220 (101.5605, 16.3919) -> (87.5555, 16.3919)
  line L221 (87.5555, 16.3919) -> (87.5555, 30.3969)
  line L222 (87.5555, 30.3969) -> (101.5605, 16.3919) construction
  line L223 (101.5605, 30.3969) -> (87.5555, 16.3919) construction
  line L224 (149.5563, 30.4305) -> (163.5613, 30.4305)
  line L225 (163.5613, 30.4305) -> (163.5613, 16.4255)
  line L226 (163.5613, 16.4255) -> (149.5563, 16.4255)
  line L227 (149.5563, 16.4255) -> (149.5563, 30.4305)
  line L228 (149.5563, 30.4305) -> (163.5613, 16.4255) construction
  line L229 (163.5613, 30.4305) -> (149.5563, 16.4255) construction
  line L230 (168.6063, 30.4305) -> (182.6113, 30.4305)
  line L231 (182.6113, 30.4305) -> (182.6113, 16.4255)
  line L232 (182.6113, 16.4255) -> (168.6063, 16.4255)
  line L233 (168.6063, 16.4255) -> (168.6063, 30.4305)
  line L234 (168.6063, 30.4305) -> (182.6113, 16.4255) construction
  line L235 (182.6113, 30.4305) -> (168.6063, 16.4255) construction
  line L236 (187.6563, 30.4305) -> (201.6613, 30.4305)
  line L237 (201.6613, 30.4305) -> (201.6613, 16.4255)
  line L238 (201.6613, 16.4255) -> (187.6563, 16.4255)
  line L239 (187.6563, 16.4255) -> (187.6563, 30.4305)
  line L240 (187.6563, 30.4305) -> (201.6613, 16.4255) construction
  line L241 (201.6613, 30.4305) -> (187.6563, 16.4255) construction
  line L242 (220.7113, 30.4305) -> (206.7063, 30.4305)
  line L243 (206.7063, 30.4305) -> (206.7063, 16.4255)
  line L244 (206.7063, 16.4255) -> (220.7113, 16.4255)
  line L245 (220.7113, 16.4255) -> (220.7113, 30.4305)
  line L246 (220.7113, 30.4305) -> (206.7063, 16.4255) construction
  line L247 (206.7063, 30.4305) -> (220.7113, 16.4255) construction
  line L248 (149.5563, 11.3805) -> (163.5613, 11.3805)
  line L249 (163.5613, 11.3805) -> (163.5613, -2.6245)
  line L250 (163.5613, -2.6245) -> (149.5563, -2.6245)
  line L251 (149.5563, -2.6245) -> (149.5563, 11.3805)
  line L252 (149.5563, 11.3805) -> (163.5613, -2.6245) construction
  line L253 (163.5613, 11.3805) -> (149.5563, -2.6245) construction
  line L254 (168.6063, 11.3805) -> (182.6113, 11.3805)
  line L255 (182.6113, 11.3805) -> (182.6113, -2.6245)
  line L256 (182.6113, -2.6245) -> (168.6063, -2.6245)
  line L257 (168.6063, -2.6245) -> (168.6063, 11.3805)
  line L258 (168.6063, 11.3805) -> (182.6113, -2.6245) construction
  line L259 (182.6113, 11.3805) -> (168.6063, -2.6245) construction
  line L260 (187.6563, 11.3805) -> (201.6613, 11.3805)
  line L261 (201.6613, 11.3805) -> (201.6613, -2.6245)
  line L262 (201.6613, -2.6245) -> (187.6563, -2.6245)
  line L263 (187.6563, -2.6245) -> (187.6563, 11.3805)
  line L264 (187.6563, 11.3805) -> (201.6613, -2.6245) construction
  line L265 (201.6613, 11.3805) -> (187.6563, -2.6245) construction
  line L266 (220.7113, 11.3805) -> (206.7063, 11.3805)
  line L267 (206.7063, 11.3805) -> (206.7063, -2.6245)
  line L268 (206.7063, -2.6245) -> (220.7113, -2.6245)
  line L269 (220.7113, -2.6245) -> (220.7113, 11.3805)
  line L270 (220.7113, 11.3805) -> (206.7063, -2.6245) construction
  line L271 (206.7063, 11.3805) -> (220.7113, -2.6245) construction
  line L272 (149.5563, -7.6695) -> (163.5613, -7.6695)
  line L273 (163.5613, -7.6695) -> (163.5613, -21.6745)
  line L274 (163.5613, -21.6745) -> (149.5563, -21.6745)
  line L275 (149.5563, -21.6745) -> (149.5563, -7.6695)
  line L276 (149.5563, -7.6695) -> (163.5613, -21.6745) construction
  line L277 (163.5613, -7.6695) -> (149.5563, -21.6745) construction
  line L278 (168.6063, -7.6695) -> (182.6113, -7.6695)
  line L279 (182.6113, -7.6695) -> (182.6113, -21.6745)
  line L280 (182.6113, -21.6745) -> (168.6063, -21.6745)
  line L281 (168.6063, -21.6745) -> (168.6063, -7.6695)
  line L282 (168.6063, -7.6695) -> (182.6113, -21.6745) construction
  line L283 (182.6113, -7.6695) -> (168.6063, -21.6745) construction
  line L284 (187.6563, -7.6695) -> (201.6613, -7.6695)
  line L285 (201.6613, -7.6695) -> (201.6613, -21.6745)
  line L286 (201.6613, -21.6745) -> (187.6563, -21.6745)
  line L287 (187.6563, -21.6745) -> (187.6563, -7.6695)
  line L288 (187.6563, -7.6695) -> (201.6613, -21.6745) construction
  line L289 (201.6613, -7.6695) -> (187.6563, -21.6745) construction
  line L290 (206.7063, -7.6695) -> (220.7113, -7.6695)
  line L291 (220.7113, -7.6695) -> (220.7113, -21.6745)
  line L292 (220.7113, -21.6745) -> (206.7063, -21.6745)
  line L293 (206.7063, -21.6745) -> (206.7063, -7.6695)
  line L294 (206.7063, -7.6695) -> (220.7113, -21.6745) construction
  line L295 (220.7113, -7.6695) -> (206.7063, -21.6745) construction
  line L296 (163.5613, -26.7195) -> (149.5563, -26.7195)
  line L297 (149.5563, -26.7195) -> (149.5563, -40.7245)
  line L298 (149.5563, -40.7245) -> (163.5613, -40.7245)
  line L299 (163.5613, -40.7245) -> (163.5613, -26.7195)
  line L300 (163.5613, -26.7195) -> (149.5563, -40.7245) construction
  line L301 (149.5563, -26.7195) -> (163.5613, -40.7245) construction
  line L302 (182.6113, -40.7245) -> (168.6063, -40.7245)
  line L303 (168.6063, -40.7245) -> (168.6063, -26.7195)
  line L304 (168.6063, -26.7195) -> (182.6113, -26.7195)
  line L305 (182.6113, -26.7195) -> (182.6113, -40.7245)
  line L306 (182.6113, -40.7245) -> (168.6063, -26.7195) construction
  line L307 (168.6063, -40.7245) -> (182.6113, -26.7195) construction
  line L308 (201.6613, -26.7195) -> (187.6563, -26.7195)
  line L309 (187.6563, -26.7195) -> (187.6563, -40.7245)
  line L310 (187.6563, -40.7245) -> (201.6613, -40.7245)
  line L311 (201.6613, -40.7245) -> (201.6613, -26.7195)
  line L312 (201.6613, -26.7195) -> (187.6563, -40.7245) construction
  line L313 (187.6563, -26.7195) -> (201.6613, -40.7245) construction
  line L314 (206.7063, -36.2715) -> (220.7113, -36.2715)
  line L315 (220.7113, -36.2715) -> (220.7113, -50.2765)
  line L316 (220.7113, -50.2765) -> (206.7063, -50.2765)
  line L317 (206.7063, -50.2765) -> (206.7063, -36.2715)
  line L318 (206.7063, -36.2715) -> (220.7113, -50.2765) construction
  line L319 (220.7113, -36.2715) -> (206.7063, -50.2765) construction
  line L320 (187.6563, -45.7695) -> (201.6613, -45.7695)
  line L321 (201.6613, -45.7695) -> (201.6613, -59.7745)
  line L322 (201.6613, -59.7745) -> (187.6563, -59.7745)
  line L323 (187.6563, -59.7745) -> (187.6563, -45.7695)
  line L324 (187.6563, -45.7695) -> (201.6613, -59.7745) construction
  line L325 (201.6613, -45.7695) -> (187.6563, -59.7745) construction
  line L326 (159.2083, -45.7695) -> (173.2133, -45.7695)
  line L327 (173.2133, -45.7695) -> (173.2133, -59.7745)
  line L328 (173.2133, -59.7745) -> (159.2083, -59.7745)
  line L329 (159.2083, -59.7745) -> (159.2083, -45.7695)
  line L330 (159.2083, -45.7695) -> (173.2133, -59.7745) construction
  line L331 (173.2133, -45.7695) -> (159.2083, -59.7745) construction
  arc A100 (222.1338, -22.3912) -> (222.1338, -26.6088) centre (220, -24.5) ccw
  line L332 (30.4468, -26.8179) -> (36.4468, -26.8179)
  line L333 (36.4468, -26.8179) -> (36.4468, -39.2179)
  line L334 (36.4468, -39.2179) -> (30.4468, -39.2179)
  line L335 (30.4468, -39.2179) -> (30.4468, -26.8179)
  line L336 (54.4468, -26.8179) -> (60.4468, -26.8179)
  line L337 (60.4468, -26.8179) -> (60.4468, -39.2179)
  line L338 (60.4468, -39.2179) -> (54.4468, -39.2179)
  line L339 (54.4468, -39.2179) -> (54.4468, -26.8179)
  line L340 (52.6683, 9.6276) -> (65.0683, 9.6276)
  line L341 (65.0683, 9.6276) -> (65.0683, 3.6276)
  line L342 (65.0683, 3.6276) -> (52.6683, 3.6276)
  line L343 (52.6683, 3.6276) -> (52.6683, 9.6276)
  line L344 (52.6683, -14.3724) -> (65.0683, -14.3724)
  line L345 (65.0683, -14.3724) -> (65.0683, -20.3724)
  line L346 (65.0683, -20.3724) -> (52.6683, -20.3724)
  line L347 (52.6683, -20.3724) -> (52.6683, -14.3724)
  line L348 (151.2108, -58.1695) -> (157.2108, -58.1695)
  line L349 (157.2108, -58.1695) -> (157.2108, -45.7695)
  line L350 (157.2108, -45.7695) -> (151.2108, -45.7695)
  line L351 (151.2108, -45.7695) -> (151.2108, -58.1695)
  line L352 (175.2108, -45.7695) -> (181.2108, -45.7695)
  line L353 (181.2108, -45.7695) -> (181.2108, -58.1695)
  line L354 (181.2108, -58.1695) -> (175.2108, -58.1695)
  line L355 (175.2108, -58.1695) -> (175.2108, -45.7695)
  line L356 (206.7063, -34.274) -> (219.1063, -34.274)
  line L357 (219.1063, -34.274) -> (219.1063, -28.274)
  line L358 (219.1063, -28.274) -> (206.7063, -28.274)
  line L359 (206.7063, -28.274) -> (206.7063, -34.274)
  line L360 (206.7063, -52.274) -> (219.1063, -52.274)
  line L361 (219.1063, -52.274) -> (219.1063, -58.274)
  line L362 (219.1063, -58.274) -> (206.7063, -58.274)
  line L363 (206.7063, -58.274) -> (206.7063, -52.274)
  point P0 (0, 0)
  point P1 (218.9918, -21.6745)
  point P2 (220.7113, -21.5855)
  dimension "d1" = 0.1
  dimension "d2" = 0.1
  dimension "d3" = 0.1
  dimension "d4" = 0.1
  dimension "d5" = 0.1
  dimension "d6" = 0.1
  dimension "d7" = 0.1
  dimension "d8" = 0.1
  dimension "d9" = 0.1
  dimension "d10" = 0.1
  dimension "d11" = 0.1
  dimension "d12" = 0.1
  dimension "d13" = 0.1
  dimension "d14" = 0.1
  dimension "d15" = 0.1
  dimension "d16" = 0.1
  dimension "d17" = 0.1
  dimension "d18" = 0.1
  dimension "d19" = 0.1
  dimension "d20" = 0.1
  dimension "d21" = 0.1
  dimension "d22" = 14.005
  dimension "d23" = 14.005
  dimension "d24" = 14.005
  dimension "d25" = 14.005
  dimension "d26" = 14.005
  dimension "d27" = 14.005
  dimension "d28" = 14.005
  dimension "d29" = 14.005
  dimension "d30" = 14.005
  dimension "d31" = 14.005
  dimension "d32" = 14.005
  dimension "d33" = 14.005
  dimension "d34" = 14.005
  dimension "d35" = 14.005
  dimension "d36" = 14.005
  dimension "d37" = 14.005
  dimension "d38" = 14.005
  dimension "d39" = 14.005
  dimension "d40" = 14.005
  dimension "d41" = 14.005
  dimension "d42" = 14.005
  dimension "d43" = 14.005
  dimension "d44" = 14.005
  dimension "d45" = 14.005
  dimension "d46" = 14.005
  dimension "d47" = 14.005
  dimension "d48" = 14.005
  dimension "d49" = 14.005
  dimension "d50" = 14.005
  dimension "d51" = 14.005
  dimension "d52" = 14.005
  dimension "d53" = 14.005
  dimension "d54" = 14.005
  dimension "d55" = 14.005
  dimension "d56" = 14.005
  dimension "d57" = 14.005
  dimension "d58" = 14.005
  dimension "d59" = 14.005
  dimension "d60" = 14.005
  dimension "d61" = 14.005
  dimension "d62" = 14.005
  dimension "d63" = 14.005
  dimension "d64" = 14.005
  constraints: 580 end point, 95 parallel, 76 midpoint, 66 perpendicular, 47 horizontal, 31 point on line, 8 collinear, 2 point on circle, 1 centre point, 1 coincident, 1 vertical
  measures "d1" distance between parallel lines of L63 L73
  measures "d2" distance between parallel lines of L62 L72
  measures "d3" distance between parallel lines of L71 L61
  measures "d4" distance between parallel lines of L64 L74
  measures "d5" distance between parallel lines of L60 L75
  measures "d6" distance between parallel lines of L59 L70
  measures "d7" distance between parallel lines of L69 L58
  measures "d8" distance between parallel lines of L57 L68
  measures "d9" distance between parallel lines of L56 L67
  measures "d10" distance between parallel lines of L54 L66
  measures "d11" distance between parallel lines of L86 L74
  measures "d12" distance between parallel lines of L73 L85
  measures "d13" distance between parallel lines of L84 L72
  measures "d14" distance between parallel lines of L83 L71
  measures "d15" distance between parallel lines of L82 L75
  measures "d16" distance between parallel lines of L70 L81
  measures "d17" distance between parallel lines of L80 L69
  measures "d18" distance between parallel lines of L79 L68
  measures "d19" distance between parallel lines of L78 L67
  measures "d20" distance between parallel lines of L76 L65
  measures "d21" distance between parallel lines of L66 L77
  measures "d22" distance of L105.end L106.end
  measures "d23" distance of L104.end L105.end
  measures "d24" distance of L111.end L112.end
  measures "d25" distance of L110.end L111.end
  measures "d26" distance of L117.end L118.end
  measures "d27" distance of L116.end L117.end
  measures "d28" distance of L123.end L124.end
  measures "d29" distance of L122.end L123.end
  measures "d30" distance of L129.end L130.end
  measures "d31" distance of L128.end L129.end
  measures "d32" distance of L135.end L136.end
  measures "d33" distance of L134.end L135.end
  measures "d34" distance of L141.end L142.end